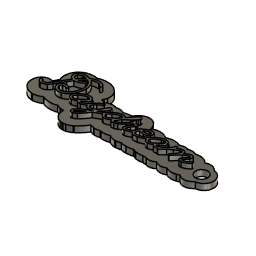
DaydreamKeyringV1 (Autodesk Fusion 360 design; units mm, degrees)
Autodesk Fusion 360 part; units mm, degrees
(part 1 of 4)
sketch "Sketch1" plane through (0, 0, 0) normal (0, 0, 1) x (1, 0, 0)
  spline S0 degree 3 poles (-17.0116, 12.697) (-15.5656, 12.5271) (-14.2829, 11.8983) (-13.2633, 10.87) knots 0 0 0 0 1 1 1 1
  line L0 (-13.2633, 10.87) -> (-13.215, 10.8207)
  line L1 (-13.215, 10.8207) -> (-13.1095, 10.7122)
  line L2 (-13.1095, 10.7122) -> (-13.0154, 10.5937)
  spline S1 degree 3 poles (-13.0154, 10.5937) (-12.1523, 9.5077) (-11.8163, 8.1682) (-12.0651, 6.8032) knots 0 0 0 0 1 1 1 1
  spline S2 degree 3 poles (-12.0651, 6.8032) (-12.1242, 6.4791) (-12.2329, 6.1392) (-12.4073, 5.8054) knots 0 0 0 0 1 1 1 1
  spline S3 degree 3 poles (-12.4073, 5.8054) (-12.5074, 5.614) (-12.6296, 5.4157) (-12.7769, 5.2205) knots 0 0 0 0 1 1 1 1
  spline S4 degree 3 poles (-12.7769, 5.2205) (-12.686, 5.1955) (-12.5953, 5.1686) (-12.505, 5.1397) knots 0 0 0 0 1 1 1 1
  spline S5 degree 3 poles (-12.505, 5.1397) (-12.3281, 5.083) (-12.1403, 5.0077) (-11.9485, 4.908) knots 0 0 0 0 1 1 1 1
  line L3 (-11.9485, 4.908) -> (-11.9101, 4.8877)
  line L4 (-11.9101, 4.8877) -> (-11.8702, 4.8661)
  spline S6 degree 3 poles (-11.8702, 4.8661) (-11.6952, 4.7703) (-11.5266, 4.6643) (-11.3653, 4.5483) knots 0 0 0 0 1 1 1 1
  spline S7 degree 3 poles (-11.3653, 4.5483) (-11.1926, 4.6617) (-11.016, 4.7697) (-10.8356, 4.8723) knots 0 0 0 0 1 1 1 1
  line L5 (-10.8356, 4.8723) -> (-10.8053, 4.8895)
  line L6 (-10.8053, 4.8895) -> (-10.7746, 4.9061)
  spline S8 degree 3 poles (-10.7746, 4.9061) (-10.3204, 5.1508) (-9.8393, 5.3371) (-9.3365, 5.4613) knots 0 0 0 0 1 1 1 1
  line L7 (-9.3365, 5.4613) -> (-9.2942, 5.4714)
  spline S9 degree 3 poles (-9.2942, 5.4714) (-8.8543, 5.5745) (-8.3289, 5.6096) (-7.7656, 5.4916) knots 0 0 0 0 1 1 1 1
  spline S10 degree 3 poles (-7.7656, 5.4916) (-7.5435, 5.4451) (-7.3065, 5.3766) (-7.0656, 5.2796) knots 0 0 0 0 1 1 1 1
  spline S11 degree 3 poles (-7.0656, 5.2796) (-7.0389, 5.2882) (-7.0121, 5.2966) (-6.985, 5.3047) knots 0 0 0 0 1 1 1 1
  spline S12 degree 3 poles (-6.985, 5.3047) (-5.8678, 5.6394) (-4.8296, 5.4328) (-4.0426, 5.0886) knots 0 0 0 0 1 1 1 1
  spline S13 degree 3 poles (-4.0426, 5.0886) (-3.921, 5.0355) (-3.7986, 4.9737) (-3.677, 4.9028) knots 0 0 0 0 1 1 1 1
  spline S14 degree 3 poles (-3.677, 4.9028) (-3.487, 4.9839) (-3.2942, 5.0598) (-3.0985, 5.1304) knots 0 0 0 0 1 1 1 1
  line L8 (-3.0985, 5.1304) -> (-3.0332, 5.1539)
  line L9 (-3.0332, 5.1539) -> (-2.9669, 5.1745)
  spline S15 degree 3 poles (-2.9669, 5.1745) (-2.2264, 5.4039) (-1.4698, 5.5072) (-0.7109, 5.4834) knots 0 0 0 0 1 1 1 1
  spline S16 degree 3 poles (-0.7109, 5.4834) (-0.4568, 5.8048) (-0.1999, 6.1247) (0.0598, 6.4431) knots 0 0 0 0 1 1 1 1
  line L10 (0.0598, 6.4431) -> (0.1573, 6.5627)
  line L11 (0.1573, 6.5627) -> (0.5924, 6.9978)
  spline S17 degree 3 poles (0.5924, 6.9978) (0.7011, 7.1065) (0.8098, 7.2152) (0.9184, 7.3239) knots 0 0 0 0 1 1 1 1
  line L12 (0.9184, 7.3239) -> (0.9577, 7.3625)
  spline S18 degree 3 poles (0.9577, 7.3625) (1.1579, 7.5569) (1.4187, 7.7663) (1.7475, 7.945) knots 0 0 0 0 1 1 1 1
  spline S19 degree 3 poles (1.7475, 7.945) (2.4822, 8.3441) (3.5755, 8.7007) (4.8203, 8.3805) knots 0 0 0 0 1 1 1 1
  spline S20 degree 3 poles (4.8203, 8.3805) (6.0538, 8.0631) (6.8371, 7.2358) (7.2909, 6.5213) knots 0 0 0 0 1 1 1 1
  line L13 (7.2909, 6.5213) -> (7.312, 6.4874)
  line L14 (7.312, 6.4874) -> (7.3319, 6.4552)
  spline S21 degree 3 poles (7.3319, 6.4552) (7.5348, 6.1216) (7.6785, 5.7617) (7.7621, 5.3924) knots 0 0 0 0 1 1 1 1
  spline S22 degree 3 poles (7.7621, 5.3924) (7.8023, 5.2143) (7.8335, 5.0337) (7.8558, 4.8512) knots 0 0 0 0 1 1 1 1
  spline S23 degree 3 poles (7.8558, 4.8512) (8.4135, 5.1588) (9.0085, 5.3986) (9.6347, 5.5692) knots 0 0 0 0 1 1 1 1
  line L15 (9.6347, 5.5692) -> (9.672, 5.5794)
  line L16 (9.672, 5.5794) -> (9.7098, 5.5886)
  spline S24 degree 3 poles (9.7098, 5.5886) (11.293, 5.9769) (12.8633, 5.6981) (14.1702, 4.7588) knots 0 0 0 0 1 1 1 1
  spline S25 degree 3 poles (14.1702, 4.7588) (14.6637, 4.9752) (15.1775, 5.1532) (15.7108, 5.2928) knots 0 0 0 0 1 1 1 1
  line L17 (15.7108, 5.2928) -> (15.8313, 5.3244)
  line L18 (15.8313, 5.3244) -> (15.9543, 5.346)
  spline S26 degree 3 poles (15.9543, 5.346) (16.9738, 5.5254) (17.9994, 5.4769) (18.9978, 5.2007) knots 0 0 0 0 1 1 1 1
  line L19 (18.9978, 5.2007) -> (19.1642, 5.1546)
  line L20 (19.1642, 5.1546) -> (19.3246, 5.0901)
  spline S27 degree 3 poles (19.3246, 5.0901) (19.4966, 5.0207) (19.6659, 4.9416) (19.8311, 4.8523) knots 0 0 0 0 1 1 1 1
  spline S28 degree 3 poles (19.8311, 4.8523) (20.051, 4.9869) (20.295, 5.1043) (20.5645, 5.1964) knots 0 0 0 0 1 1 1 1
  spline S29 degree 3 poles (20.5645, 5.1964) (21.4931, 5.5135) (22.3624, 5.406) (23.0154, 5.1941) knots 0 0 0 0 1 1 1 1
  spline S30 degree 3 poles (23.0154, 5.1941) (23.3835, 5.2965) (23.7594, 5.3726) (24.1417, 5.422) knots 0 0 0 0 1 1 1 1
  line L21 (24.1417, 5.422) -> (24.1774, 5.4264)
  spline S31 degree 3 poles (24.1774, 5.4264) (24.3442, 5.4463) (24.5277, 5.4565) (24.7241, 5.4497) knots 0 0 0 0 1 1 1 1
  line L22 (24.7241, 5.4497) -> (24.7663, 5.448)
  line L23 (24.7663, 5.448) -> (24.8398, 5.4441)
  spline S32 degree 3 poles (24.8398, 5.4441) (25.3605, 5.4125) (25.9124, 5.2986) (26.451, 5.0601) knots 0 0 0 0 1 1 1 1
  spline S33 degree 3 poles (26.451, 5.0601) (27.0557, 5.231) (27.6787, 5.313) (28.3094, 5.3117) knots 0 0 0 0 1 1 1 1
  line L24 (28.3094, 5.3117) -> (28.365, 5.3111)
  spline S34 degree 3 poles (28.365, 5.3111) (28.626, 5.3065) (28.8951, 5.2734) (29.1654, 5.2065) knots 0 0 0 0 1 1 1 1
  line L25 (29.1654, 5.2065) -> (29.223, 5.1916)
  line L26 (29.223, 5.1916) -> (29.2681, 5.1795)
  spline S35 degree 3 poles (29.2681, 5.1795) (30.2162, 4.9191) (31.3201, 4.3441) (32.0218, 3.1648) knots 0 0 0 0 1 1 1 1
  spline S36 degree 3 poles (32.0218, 3.1648) (32.1022, 3.0293) (32.1732, 2.8929) (32.2357, 2.7561) knots 0 0 0 0 1 1 1 1
  spline S37 degree 3 poles (32.2357, 2.7561) (32.8128, 2.5092) (33.2719, 2.1383) (33.616, 1.7489) knots 0 0 0 0 1 1 1 1
  line L27 (33.616, 1.7489) -> (33.6619, 1.6961)
  line L28 (33.6619, 1.6961) -> (33.6935, 1.6581)
  spline S38 degree 3 poles (33.6935, 1.6581) (34.3563, 0.8587) (34.502, -0.0325) (34.502, -0.6217) knots 0 0 0 0 1 1 1 1
  line L29 (34.502, -0.6217) -> (34.502, -1.0976)
  spline S39 degree 3 poles (34.502, -1.0976) (34.502, -1.9144) (34.2285, -2.775) (33.6258, -3.4796) knots 0 0 0 0 1 1 1 1
  spline S40 degree 3 poles (33.6258, -3.4796) (32.549, -4.7372) (31.2024, -5.649) (29.6415, -6.2002) knots 0 0 0 0 1 1 1 1
  spline S41 degree 3 poles (29.6415, -6.2002) (29.639, -6.2011) (29.6366, -6.202) (29.6338, -6.2029) knots 0 0 0 0 1 1 1 1
  spline S42 degree 3 poles (29.6338, -6.2029) (29.6313, -6.2038) (29.6285, -6.2048) (29.6256, -6.2058) knots 0 0 0 0 1 1 1 1
  spline S43 degree 3 poles (29.6256, -6.2058) (28.2575, -6.6903) (26.8147, -6.6195) (25.4936, -5.9673) knots 0 0 0 0 1 1 1 1
  spline S44 degree 3 poles (25.4936, -5.9673) (25.4542, -5.9479) (25.4145, -5.9271) (25.3735, -5.9051) knots 0 0 0 0 1 1 1 1
  spline S45 degree 3 poles (25.3735, -5.9051) (24.125, -6.7788) (22.3924, -6.8462) (21.058, -5.8602) knots 0 0 0 0 1 1 1 1
  spline S46 degree 3 poles (21.058, -5.8602) (20.2146, -6.6354) (18.8116, -7.0734) (17.5047, -6.5966) knots 0 0 0 0 1 1 1 1
  line L30 (17.5047, -6.5966) -> (17.4605, -6.5984)
  spline S47 degree 3 poles (17.4605, -6.5984) (16.9726, -6.6187) (16.4758, -6.5698) (15.9868, -6.438) knots 0 0 0 0 1 1 1 1
  spline S48 degree 3 poles (15.9868, -6.438) (15.0484, -6.7163) (14.0736, -6.7516) (13.1093, -6.5671) knots 0 0 0 0 1 1 1 1
  line L31 (13.1093, -6.5671) -> (12.9761, -6.5416)
  line L32 (12.9761, -6.5416) -> (12.8455, -6.5043)
  spline S49 degree 3 poles (12.8455, -6.5043) (12.5062, -6.4075) (12.1742, -6.277) (11.8556, -6.1104) knots 0 0 0 0 1 1 1 1
  spline S50 degree 3 poles (11.8556, -6.1104) (10.959, -6.4139) (10.0264, -6.5894) (9.0657, -6.6378) knots 0 0 0 0 1 1 1 1
  spline S51 degree 3 poles (9.0657, -6.6378) (8.3392, -6.6769) (7.6135, -6.5812) (6.922, -6.3326) knots 0 0 0 0 1 1 1 1
  spline S52 degree 3 poles (6.922, -6.3326) (6.2803, -6.5562) (5.6161, -6.707) (4.9338, -6.7845) knots 0 0 0 0 1 1 1 1
  line L33 (4.9338, -6.7845) -> (4.7783, -6.8022)
  line L34 (4.7783, -6.8022) -> (4.6218, -6.8038)
  spline S53 degree 3 poles (4.6218, -6.8038) (3.8027, -6.8123) (2.8406, -6.6275) (1.968, -6.0062) knots 0 0 0 0 1 1 1 1
  spline S54 degree 3 poles (1.968, -6.0062) (1.9586, -5.9996) (1.9493, -5.9928) (1.9401, -5.9861) knots 0 0 0 0 1 1 1 1
  spline S55 degree 3 poles (1.9401, -5.9861) (0.8662, -6.4685) (-0.2935, -6.6357) (-1.4742, -6.47) knots 0 0 0 0 1 1 1 1
  line L35 (-1.4742, -6.47) -> (-1.6858, -6.4404)
  line L36 (-1.6858, -6.4404) -> (-1.8911, -6.3814)
  spline S56 degree 3 poles (-1.8911, -6.3814) (-1.8936, -6.3807) (-1.8961, -6.38) (-1.8986, -6.3792) knots 0 0 0 0 1 1 1 1
  spline S57 degree 3 poles (-1.8986, -6.3792) (-2.6487, -6.6088) (-3.4266, -6.6988) (-4.213, -6.6578) knots 0 0 0 0 1 1 1 1
  line L37 (-4.213, -6.6578) -> (-4.3, -6.6533)
  line L38 (-4.3, -6.6533) -> (-4.3865, -6.6438)
  spline S58 degree 3 poles (-4.3865, -6.6438) (-4.8971, -6.5878) (-5.4048, -6.461) (-5.8897, -6.2522) knots 0 0 0 0 1 1 1 1
  spline S59 degree 3 poles (-5.8897, -6.2522) (-5.897, -6.2561) (-5.9044, -6.2599) (-5.9117, -6.2637) knots 0 0 0 0 1 1 1 1
  spline S60 degree 3 poles (-5.9117, -6.2637) (-6.8039, -7.6764) (-7.8863, -8.94) (-9.1522, -10.0482) knots 0 0 0 0 1 1 1 1
  line L39 (-9.1522, -10.0482) -> (-9.2488, -10.1326)
  line L40 (-9.2488, -10.1326) -> (-9.352, -10.2087)
  spline S61 degree 3 poles (-9.352, -10.2087) (-9.9808, -10.6718) (-10.6783, -11.0211) (-11.4328, -11.2431) knots 0 0 0 0 1 1 1 1
  spline S62 degree 3 poles (-11.4328, -11.2431) (-11.7998, -11.3511) (-12.1496, -11.3902) (-12.4606, -11.3902) knots 0 0 0 0 1 1 1 1
  line L41 (-12.4606, -11.3902) -> (-12.8404, -11.3902)
  spline S63 degree 3 poles (-12.8404, -11.3902) (-13.0495, -11.3902) (-13.3343, -11.3729) (-13.6596, -11.2964) knots 0 0 0 0 1 1 1 1
  spline S64 degree 3 poles (-13.6596, -11.2964) (-14.941, -10.9952) (-15.9537, -10.1675) (-16.5217, -9.0129) knots 0 0 0 0 1 1 1 1
  spline S65 degree 3 poles (-16.5217, -9.0129) (-16.6574, -8.7371) (-16.7448, -8.4674) (-16.7998, -8.221) knots 0 0 0 0 1 1 1 1
  spline S66 degree 3 poles (-16.7998, -8.221) (-16.9174, -7.6941) (-16.9595, -7.1724) (-16.9287, -6.6644) knots 0 0 0 0 1 1 1 1
  spline S67 degree 3 poles (-16.9287, -6.6644) (-17.3371, -6.6975) (-17.7496, -6.6895) (-18.1624, -6.6418) knots 0 0 0 0 1 1 1 1
  line L42 (-18.1624, -6.6418) -> (-18.2993, -6.626)
  line L43 (-18.2993, -6.626) -> (-18.4342, -6.5979)
  spline S68 degree 3 poles (-18.4342, -6.5979) (-18.9423, -6.492) (-19.4621, -6.3149) (-19.9578, -6.0404) knots 0 0 0 0 1 1 1 1
  spline S69 degree 3 poles (-19.9578, -6.0404) (-21.8163, -6.8437) (-23.8226, -6.7614) (-25.7467, -6.0039) knots 0 0 0 0 1 1 1 1
  line L44 (-25.7467, -6.0039) -> (-25.9385, -5.9284)
  line L45 (-25.9385, -5.9284) -> (-26.0235, -5.8808)
  spline S70 degree 3 poles (-26.0235, -5.8808) (-27.0239, -6.612) (-28.1898, -7.0211) (-29.451, -7.0843) knots 0 0 0 0 1 1 1 1
  line L46 (-29.451, -7.0843) -> (-29.618, -7.0926)
  line L47 (-29.618, -7.0926) -> (-29.7849, -7.0826)
  spline S71 degree 3 poles (-29.7849, -7.0826) (-31.5585, -6.9767) (-33.0924, -6.1128) (-34.0693, -4.5827) knots 0 0 0 0 1 1 1 1
  spline S72 degree 3 poles (-34.0693, -4.5827) (-34.2876, -4.2408) (-34.4452, -3.8656) (-34.537, -3.4741) knots 0 0 0 0 1 1 1 1
  spline S73 degree 3 poles (-34.537, -3.4741) (-34.6825, -2.854) (-34.729, -2.2215) (-34.6769, -1.5881) knots 0 0 0 0 1 1 1 1
  spline S74 degree 3 poles (-34.6769, -1.5881) (-34.6399, -1.1377) (-34.5131, -0.6391) (-34.2428, -0.1539) knots 0 0 0 0 1 1 1 1
  line L48 (-34.2428, -0.1539) -> (-34.2072, -0.0914)
  spline S75 degree 3 poles (-34.2072, -0.0914) (-33.8311, 0.5581) (-33.1666, 1.3164) (-32.0873, 1.6748) knots 0 0 0 0 1 1 1 1
  spline S76 degree 3 poles (-32.0873, 1.6748) (-31.2617, 1.949) (-30.4923, 1.8894) (-29.8752, 1.722) knots 0 0 0 0 1 1 1 1
  spline S77 degree 3 poles (-29.8752, 1.722) (-29.538, 2.3142) (-29.2125, 2.914) (-28.8989, 3.5214) knots 0 0 0 0 1 1 1 1
  line L49 (-28.8989, 3.5214) -> (-28.8667, 3.5837)
  line L50 (-28.8667, 3.5837) -> (-28.8316, 3.6446)
  spline S78 degree 3 poles (-28.8316, 3.6446) (-28.8105, 3.6813) (-28.7892, 3.718) (-28.768, 3.7547) knots 0 0 0 0 1 1 1 1
  spline S79 degree 3 poles (-28.768, 3.7547) (-28.8892, 3.9964) (-28.9939, 4.2524) (-29.0788, 4.5231) knots 0 0 0 0 1 1 1 1
  spline S80 degree 3 poles (-29.0788, 4.5231) (-29.4617, 5.7423) (-29.3472, 6.9455) (-29.015, 7.995) knots 0 0 0 0 1 1 1 1
  line L51 (-29.015, 7.995) -> (-28.9707, 8.1349)
  line L52 (-28.9707, 8.1349) -> (-28.9131, 8.2699)
  spline S81 degree 3 poles (-28.9131, 8.2699) (-28.4879, 9.2675) (-27.8342, 10.1832) (-26.8945, 10.8753) knots 0 0 0 0 1 1 1 1
  spline S82 degree 3 poles (-26.8945, 10.8753) (-25.9553, 11.5669) (-24.8876, 11.9194) (-23.8109, 12.0317) knots 0 0 0 0 1 1 1 1
  line L53 (-23.8109, 12.0317) -> (-23.8069, 12.0321)
  line L54 (-23.8069, 12.0321) -> (-23.8029, 12.0325)
  spline S83 degree 3 poles (-23.8029, 12.0325) (-23.0183, 12.1123) (-22.2378, 12.0846) (-21.4699, 11.9478) knots 0 0 0 0 1 1 1 1
  spline S84 degree 3 poles (-21.4699, 11.9478) (-20.7386, 12.2804) (-19.9708, 12.519) (-19.1721, 12.6612) knots 0 0 0 0 1 1 1 1
  line L55 (-19.1721, 12.6612) -> (-19.1303, 12.6684)
  spline S85 degree 3 poles (-19.1303, 12.6684) (-18.9214, 12.7031) (-18.7199, 12.7178) (-18.5296, 12.7178) knots 0 0 0 0 1 1 1 1
  line L56 (-18.5296, 12.7178) -> (-17.1886, 12.7178)
  line L57 (-17.1886, 12.7178) -> (-17.0116, 12.697)
  spline S86 degree 3 poles (-18.5843, 9.6739) (-18.1785, 9.6739) (-17.7726, 9.6739) (-17.3668, 9.6739) knots 0 0 0 0 1 1 1 1
  spline S87 degree 3 poles (-17.3668, 9.6739) (-16.5975, 9.5835) (-15.9414, 9.2588) (-15.3984, 8.6998) knots 0 0 0 0 1 1 1 1
  spline S88 degree 3 poles (-15.3984, 8.6998) (-15.0666, 8.2823) (-14.9583, 7.8088) (-15.0737, 7.2793) knots 0 0 0 0 1 1 1 1
  spline S89 degree 3 poles (-15.0737, 7.2793) (-15.2904, 6.8099) (-15.6489, 6.6543) (-16.1492, 6.8126) knots 0 0 0 0 1 1 1 1
  spline S90 degree 3 poles (-16.1492, 6.8126) (-16.2169, 6.8531) (-16.2845, 6.8937) (-16.3521, 6.9343) knots 0 0 0 0 1 1 1 1
  spline S91 degree 3 poles (-16.3521, 6.9343) (-16.4811, 7.1516) (-16.6299, 7.3546) (-16.7986, 7.5431) knots 0 0 0 0 1 1 1 1
  spline S92 degree 3 poles (-16.7986, 7.5431) (-17.3698, 7.8024) (-17.965, 7.87) (-18.5843, 7.746) knots 0 0 0 0 1 1 1 1
  spline S93 degree 3 poles (-18.5843, 7.746) (-18.7718, 7.7229) (-18.9476, 7.6688) (-19.112, 7.5837) knots 0 0 0 0 1 1 1 1
  spline S94 degree 3 poles (-19.112, 7.5837) (-18.2215, 6.7294) (-17.7142, 5.6809) (-17.59, 4.4383) knots 0 0 0 0 1 1 1 1
  spline S95 degree 3 poles (-17.59, 4.4383) (-17.5629, 3.8295) (-17.5629, 3.2207) (-17.59, 2.6119) knots 0 0 0 0 1 1 1 1
  spline S96 degree 3 poles (-17.59, 2.6119) (-17.6592, 2.0632) (-17.7539, 1.522) (-17.8741, 0.9885) knots 0 0 0 0 1 1 1 1
  spline S97 degree 3 poles (-17.8741, 0.9885) (-17.0334, 1.7098) (-16.0662, 2.1765) (-14.9722, 2.3887) knots 0 0 0 0 1 1 1 1
  spline S98 degree 3 poles (-14.9722, 2.3887) (-14.4313, 2.4525) (-13.9037, 2.3984) (-13.3894, 2.2264) knots 0 0 0 0 1 1 1 1
  spline S99 degree 3 poles (-13.3894, 2.2264) (-12.9647, 2.0117) (-12.6806, 1.6802) (-12.5371, 1.232) knots 0 0 0 0 1 1 1 1
  spline S100 degree 3 poles (-12.5371, 1.232) (-11.793, 1.252) (-11.4615, 0.8867) (-11.5427, 0.1362) knots 0 0 0 0 1 1 1 1
  spline S101 degree 3 poles (-11.5427, 0.1362) (-10.9777, 1.0123) (-10.2404, 1.7091) (-9.3308, 2.2264) knots 0 0 0 0 1 1 1 1
  spline S102 degree 3 poles (-9.3308, 2.2264) (-9.0677, 2.3681) (-8.7903, 2.4696) (-8.4988, 2.5308) knots 0 0 0 0 1 1 1 1
  spline S103 degree 3 poles (-8.4988, 2.5308) (-7.9663, 2.4609) (-7.716, 2.1565) (-7.7479, 1.6176) knots 0 0 0 0 1 1 1 1
  spline S104 degree 3 poles (-7.7479, 1.6176) (-7.7057, 1.3519) (-7.7733, 1.1219) (-7.9509, 0.9276) knots 0 0 0 0 1 1 1 1
  spline S105 degree 3 poles (-7.9509, 0.9276) (-7.9323, 0.9108) (-7.9188, 0.8905) (-7.9103, 0.8667) knots 0 0 0 0 1 1 1 1
  spline S106 degree 3 poles (-7.9103, 0.8667) (-9.1699, 0.4067) (-10.0763, -0.4321) (-10.6295, -1.6496) knots 0 0 0 0 1 1 1 1
  spline S107 degree 3 poles (-10.6295, -1.6496) (-10.5539, -1.7102) (-10.466, -1.7372) (-10.3657, -1.7308) knots 0 0 0 0 1 1 1 1
  spline S108 degree 3 poles (-10.3657, -1.7308) (-9.521, -1.5488) (-8.777, -1.1701) (-8.1335, -0.5943) knots 0 0 0 0 1 1 1 1
  spline S109 degree 3 poles (-8.1335, -0.5943) (-7.6871, 0.2174) (-7.2406, 1.0291) (-6.7942, 1.8408) knots 0 0 0 0 1 1 1 1
  spline S110 degree 3 poles (-6.7942, 1.8408) (-6.3791, 2.4405) (-5.8447, 2.5825) (-5.191, 2.2669) knots 0 0 0 0 1 1 1 1
  spline S111 degree 3 poles (-5.191, 2.2669) (-4.8735, 2.0049) (-4.7383, 1.6667) (-4.7852, 1.2523) knots 0 0 0 0 1 1 1 1
  spline S112 degree 3 poles (-4.7852, 1.2523) (-4.7831, 0.9799) (-4.817, 0.716) (-4.8866, 0.4609) knots 0 0 0 0 1 1 1 1
  spline S113 degree 3 poles (-4.8866, 0.4609) (-4.0846, 1.276) (-3.1443, 1.8781) (-2.0659, 2.2669) knots 0 0 0 0 1 1 1 1
  spline S114 degree 3 poles (-2.0659, 2.2669) (-1.4097, 2.4703) (-0.7468, 2.4974) (-0.0772, 2.3481) knots 0 0 0 0 1 1 1 1
  spline S115 degree 3 poles (-0.0772, 2.3481) (0.1305, 2.2835) (0.3267, 2.1956) (0.5113, 2.0843) knots 0 0 0 0 1 1 1 1
  spline S116 degree 3 poles (0.5113, 2.0843) (1.1286, 2.9052) (1.7644, 3.717) (2.4188, 4.5195) knots 0 0 0 0 1 1 1 1
  spline S117 degree 3 poles (2.4188, 4.5195) (2.6555, 4.7562) (2.8923, 4.993) (3.1291, 5.2297) knots 0 0 0 0 1 1 1 1
  spline S118 degree 3 poles (3.1291, 5.2297) (3.8271, 5.6416) (4.375, 5.4996) (4.7728, 4.8036) knots 0 0 0 0 1 1 1 1
  spline S119 degree 3 poles (4.7728, 4.8036) (4.9427, 4.1562) (4.8277, 3.5677) (4.4278, 3.0381) knots 0 0 0 0 1 1 1 1
  spline S120 degree 3 poles (4.4278, 3.0381) (4.8861, 2.8843) (5.116, 2.5664) (5.1178, 2.0843) knots 0 0 0 0 1 1 1 1
  spline S121 degree 3 poles (5.1178, 2.0843) (6.2434, 2.0747) (6.6829, 1.52) (6.437, 0.4203) knots 0 0 0 0 1 1 1 1
  spline S122 degree 3 poles (6.437, 0.4203) (6.3939, 0.2937) (6.3395, 0.172) (6.2746, 0.055) knots 0 0 0 0 1 1 1 1
  spline S123 degree 3 poles (6.2746, 0.055) (5.8316, -0.5466) (5.3986, -1.1554) (4.9757, -1.7713) knots 0 0 0 0 1 1 1 1
  spline S124 degree 3 poles (4.9757, -1.7713) (4.9582, -1.816) (4.9785, -1.8431) (5.0366, -1.8525) knots 0 0 0 0 1 1 1 1
  spline S125 degree 3 poles (5.0366, -1.8525) (5.6366, -1.6472) (6.2048, -1.3766) (6.7413, -1.0408) knots 0 0 0 0 1 1 1 1
  spline S126 degree 3 poles (6.7413, -1.0408) (6.8229, -0.6267) (6.965, -0.2344) (7.1675, 0.1362) knots 0 0 0 0 1 1 1 1
  spline S127 degree 3 poles (7.1675, 0.1362) (7.0741, 0.9093) (7.4191, 1.3084) (8.2024, 1.3335) knots 0 0 0 0 1 1 1 1
  spline S128 degree 3 poles (8.2024, 1.3335) (8.8283, 1.9645) (9.5726, 2.3974) (10.4347, 2.6322) knots 0 0 0 0 1 1 1 1
  spline S129 degree 3 poles (10.4347, 2.6322) (11.2987, 2.8441) (12.0496, 2.6479) (12.6872, 2.0437) knots 0 0 0 0 1 1 1 1
  spline S130 degree 3 poles (12.6872, 2.0437) (12.9575, 1.665) (13.0727, 1.2456) (13.0321, 0.7856) knots 0 0 0 0 1 1 1 1
  spline S131 degree 3 poles (13.0321, 0.7856) (13.0017, 0.5473) (12.9542, 0.3173) (12.8901, 0.0956) knots 0 0 0 0 1 1 1 1
  spline S132 degree 3 poles (12.8901, 0.0956) (13.8483, 1.2211) (15.0456, 1.972) (16.4819, 2.3481) knots 0 0 0 0 1 1 1 1
  spline S133 degree 3 poles (16.4819, 2.3481) (17.057, 2.4493) (17.6252, 2.4222) (18.1865, 2.2669) knots 0 0 0 0 1 1 1 1
  spline S134 degree 3 poles (18.1865, 2.2669) (18.674, 2.0704) (18.9987, 1.7255) (19.1606, 1.232) knots 0 0 0 0 1 1 1 1
  spline S135 degree 3 poles (19.1606, 1.232) (19.6371, 1.3023) (19.9553, 1.1129) (20.1144, 0.6638) knots 0 0 0 0 1 1 1 1
  spline S136 degree 3 poles (20.1144, 0.6638) (20.1278, 0.4744) (20.1416, 0.285) (20.1549, 0.0956) knots 0 0 0 0 1 1 1 1
  spline S137 degree 3 poles (20.1549, 0.0956) (20.4545, 0.4356) (20.7386, 0.7874) (21.0072, 1.1508) knots 0 0 0 0 1 1 1 1
  spline S138 degree 3 poles (21.0072, 1.1508) (21.0129, 1.3976) (21.0397, 1.6412) (21.0884, 1.8814) knots 0 0 0 0 1 1 1 1
  spline S139 degree 3 poles (21.0884, 1.8814) (21.3315, 2.3279) (21.6899, 2.4564) (22.1639, 2.2669) knots 0 0 0 0 1 1 1 1
  spline S140 degree 3 poles (22.1639, 2.2669) (22.252, 2.2061) (22.3397, 2.1452) (22.4278, 2.0843) knots 0 0 0 0 1 1 1 1
  spline S141 degree 3 poles (22.4278, 2.0843) (22.4927, 1.9675) (22.567, 1.8593) (22.651, 1.7596) knots 0 0 0 0 1 1 1 1
  spline S142 degree 3 poles (22.651, 1.7596) (23.2488, 2.11) (23.8913, 2.3264) (24.5788, 2.409) knots 0 0 0 0 1 1 1 1
  spline S143 degree 3 poles (24.5788, 2.409) (25.2643, 2.392) (25.7241, 2.0673) (25.9587, 1.4349) knots 0 0 0 0 1 1 1 1
  spline S144 degree 3 poles (25.9587, 1.4349) (26.6625, 2.0068) (27.4677, 2.2841) (28.3736, 2.2669) knots 0 0 0 0 1 1 1 1
  spline S145 degree 3 poles (28.3736, 2.2669) (29.3464, 2.0342) (29.732, 1.4187) (29.5303, 0.4203) knots 0 0 0 0 1 1 1 1
  spline S146 degree 3 poles (29.5303, 0.4203) (29.3549, -0.2482) (29.0371, -0.8366) (28.5765, -1.3452) knots 0 0 0 0 1 1 1 1
  spline S147 degree 3 poles (28.5765, -1.3452) (28.8456, -1.2444) (29.1025, -1.1091) (29.3476, -0.9393) knots 0 0 0 0 1 1 1 1
  spline S148 degree 3 poles (29.3476, -0.9393) (29.6707, -0.6839) (29.982, -0.4133) (30.2811, -0.1276) knots 0 0 0 0 1 1 1 1
  spline S149 degree 3 poles (30.2811, -0.1276) (30.7718, 0.1303) (31.1638, 0.0288) (31.4581, -0.432) knots 0 0 0 0 1 1 1 1
  spline S150 degree 3 poles (31.4581, -0.432) (31.4581, -0.7296) (31.4581, -1.0273) (31.4581, -1.3249) knots 0 0 0 0 1 1 1 1
  spline S151 degree 3 poles (31.4581, -1.3249) (30.7109, -2.2613) (29.764, -2.931) (28.6171, -3.3339) knots 0 0 0 0 1 1 1 1
  spline S152 degree 3 poles (28.6171, -3.3339) (27.9876, -3.5589) (27.3788, -3.5183) (26.7907, -3.2121) knots 0 0 0 0 1 1 1 1
  spline S153 degree 3 poles (26.7907, -3.2121) (26.6154, -3.0776) (26.4871, -2.9085) (26.4052, -2.7048) knots 0 0 0 0 1 1 1 1
  spline S154 degree 3 poles (26.4052, -2.7048) (26.2542, -2.0827) (26.3487, -1.501) (26.6893, -0.9596) knots 0 0 0 0 1 1 1 1
  spline S155 degree 3 poles (26.6893, -0.9596) (27.0286, -0.5461) (27.3597, -0.1267) (27.6836, 0.2985) knots 0 0 0 0 1 1 1 1
  spline S156 degree 3 poles (27.6836, 0.2985) (27.6633, 0.3121) (27.643, 0.3256) (27.6227, 0.3391) knots 0 0 0 0 1 1 1 1
  spline S157 degree 3 poles (27.6227, 0.3391) (27.098, 0.087) (26.6174, -0.2309) (26.1819, -0.6146) knots 0 0 0 0 1 1 1 1
  spline S158 degree 3 poles (26.1819, -0.6146) (25.1608, -1.6118) (24.2204, -2.6738) (23.3612, -3.8006) knots 0 0 0 0 1 1 1 1
  spline S159 degree 3 poles (23.3612, -3.8006) (22.9586, -3.4876) (22.5592, -3.1697) (22.1639, -2.8469) knots 0 0 0 0 1 1 1 1
  spline S160 degree 3 poles (22.1639, -2.8469) (22.2179, -2.7928) (22.2723, -2.7386) (22.3263, -2.6845) knots 0 0 0 0 1 1 1 1
  spline S161 degree 3 poles (22.3263, -2.6845) (22.2723, -2.6304) (22.2179, -2.5763) (22.1639, -2.5222) knots 0 0 0 0 1 1 1 1
  spline S162 degree 3 poles (22.1639, -2.5222) (22.8738, -1.7308) (23.5301, -0.8987) (24.1324, -0.0261) knots 0 0 0 0 1 1 1 1
  spline S163 degree 3 poles (24.1324, -0.0261) (24.2387, 0.1584) (24.3199, 0.3478) (24.3759, 0.5421) knots 0 0 0 0 1 1 1 1
  spline S164 degree 3 poles (24.3759, 0.5421) (23.4639, 0.1777) (22.6319, -0.3161) (21.8798, -0.9393) knots 0 0 0 0 1 1 1 1
  spline S165 degree 3 poles (21.8798, -0.9393) (21.5418, -1.2234) (21.2033, -1.5075) (20.8652, -1.7916) knots 0 0 0 0 1 1 1 1
  spline S166 degree 3 poles (20.8652, -1.7916) (20.1667, -2.5104) (19.4496, -3.2072) (18.7142, -3.8818) knots 0 0 0 0 1 1 1 1
  spline S167 degree 3 poles (18.7142, -3.8818) (18.5339, -3.7624) (18.3716, -3.6204) (18.2271, -3.4556) knots 0 0 0 0 1 1 1 1
  spline S168 degree 3 poles (18.2271, -3.4556) (17.9321, -3.491) (17.6342, -3.5248) (17.3342, -3.5571) knots 0 0 0 0 1 1 1 1
  spline S169 degree 3 poles (17.3342, -3.5571) (16.8285, -3.5781) (16.3959, -3.4158) (16.0355, -3.0701) knots 0 0 0 0 1 1 1 1
  spline S170 degree 3 poles (16.0355, -3.0701) (15.3216, -3.572) (14.5371, -3.7411) (13.6815, -3.5774) knots 0 0 0 0 1 1 1 1
  spline S171 degree 3 poles (13.6815, -3.5774) (13.0946, -3.4098) (12.6685, -3.0513) (12.4031, -2.5019) knots 0 0 0 0 1 1 1 1
  spline S172 degree 3 poles (12.4031, -2.5019) (11.3352, -3.1689) (10.1721, -3.5342) (8.9127, -3.5977) knots 0 0 0 0 1 1 1 1
  spline S173 degree 3 poles (8.9127, -3.5977) (8.1968, -3.6388) (7.588, -3.4088) (7.0863, -2.9077) knots 0 0 0 0 1 1 1 1
  spline S174 degree 3 poles (7.0863, -2.9077) (6.3148, -3.3745) (5.4828, -3.6586) (4.5901, -3.76) knots 0 0 0 0 1 1 1 1
  spline S175 degree 3 poles (4.5901, -3.76) (3.8744, -3.7675) (3.4211, -3.4293) (3.2305, -2.7454) knots 0 0 0 0 1 1 1 1
  spline S176 degree 3 poles (3.2305, -2.7454) (3.2034, -2.4207) (3.2034, -2.096) (3.2305, -1.7713) knots 0 0 0 0 1 1 1 1
  spline S177 degree 3 poles (3.2305, -1.7713) (3.2998, -1.5369) (3.3675, -1.3069) (3.4334, -1.0814) knots 0 0 0 0 1 1 1 1
  spline S178 degree 3 poles (3.4334, -1.0814) (2.705, -1.9319) (1.8459, -2.6151) (0.8562, -3.131) knots 0 0 0 0 1 1 1 1
  spline S179 degree 3 poles (0.8562, -3.131) (0.2522, -3.4411) (-0.3836, -3.5493) (-1.0513, -3.4556) knots 0 0 0 0 1 1 1 1
  spline S180 degree 3 poles (-1.0513, -3.4556) (-1.3451, -3.3713) (-1.5751, -3.2022) (-1.7412, -2.9483) knots 0 0 0 0 1 1 1 1
  spline S181 degree 3 poles (-1.7412, -2.9483) (-2.4352, -3.439) (-3.2063, -3.6622) (-4.0546, -3.618) knots 0 0 0 0 1 1 1 1
  spline S182 degree 3 poles (-4.0546, -3.618) (-4.7579, -3.5408) (-5.2787, -3.1959) (-5.6172, -2.5831) knots 0 0 0 0 1 1 1 1
  spline S183 degree 3 poles (-5.6172, -2.5831) (-6.4063, -3.0826) (-7.2247, -3.5358) (-8.0726, -3.9427) knots 0 0 0 0 1 1 1 1
  spline S184 degree 3 poles (-8.0726, -3.9427) (-8.8787, -5.3917) (-9.9069, -6.6633) (-11.1571, -7.7577) knots 0 0 0 0 1 1 1 1
  spline S185 degree 3 poles (-11.1571, -7.7577) (-11.5291, -8.0317) (-11.935, -8.2279) (-12.3747, -8.3462) knots 0 0 0 0 1 1 1 1
  spline S186 degree 3 poles (-12.3747, -8.3462) (-12.5506, -8.3462) (-12.7265, -8.3462) (-12.9023, -8.3462) knots 0 0 0 0 1 1 1 1
  spline S187 degree 3 poles (-12.9023, -8.3462) (-13.3303, -8.2638) (-13.6347, -8.0203) (-13.8155, -7.6157) knots 0 0 0 0 1 1 1 1
  spline S188 degree 3 poles (-13.8155, -7.6157) (-14.0191, -6.7795) (-13.8297, -6.049) (-13.2473, -5.4241) knots 0 0 0 0 1 1 1 1
  spline S189 degree 3 poles (-13.2473, -5.4241) (-12.546, -4.6884) (-11.7681, -4.0526) (-10.9136, -3.5165) knots 0 0 0 0 1 1 1 1
  spline S190 degree 3 poles (-10.9136, -3.5165) (-11.3951, -3.3863) (-11.774, -3.1157) (-12.05, -2.7048) knots 0 0 0 0 1 1 1 1
  spline S191 degree 3 poles (-12.05, -2.7048) (-12.7352, -3.1995) (-13.4996, -3.4836) (-14.3431, -3.5571) knots 0 0 0 0 1 1 1 1
  spline S192 degree 3 poles (-14.3431, -3.5571) (-14.8508, -3.5662) (-15.2904, -3.4038) (-15.6622, -3.0701) knots 0 0 0 0 1 1 1 1
  spline S193 degree 3 poles (-15.6622, -3.0701) (-16.3095, -3.5262) (-17.0266, -3.7088) (-17.8132, -3.618) knots 0 0 0 0 1 1 1 1
  spline S194 degree 3 poles (-17.8132, -3.618) (-18.7361, -3.4257) (-19.2705, -2.8642) (-19.4163, -1.9337) knots 0 0 0 0 1 1 1 1
  spline S195 degree 3 poles (-19.4163, -1.9337) (-20.8698, -3.5555) (-22.6083, -3.9682) (-24.6316, -3.1715) knots 0 0 0 0 1 1 1 1
  spline S196 degree 3 poles (-24.6316, -3.1715) (-25.4349, -2.7219) (-25.8881, -2.0387) (-25.9912, -1.122) knots 0 0 0 0 1 1 1 1
  spline S197 degree 3 poles (-25.9912, -1.122) (-26.3947, -1.8812) (-26.902, -2.5643) (-27.5132, -3.1715) knots 0 0 0 0 1 1 1 1
  spline S198 degree 3 poles (-27.5132, -3.1715) (-28.1026, -3.713) (-28.7993, -4.0038) (-29.6034, -4.0441) knots 0 0 0 0 1 1 1 1
  spline S199 degree 3 poles (-29.6034, -4.0441) (-30.4648, -3.9927) (-31.1141, -3.6003) (-31.5515, -2.8672) knots 0 0 0 0 1 1 1 1
  spline S200 degree 3 poles (-31.5515, -2.8672) (-31.6504, -2.4947) (-31.6775, -2.1159) (-31.6327, -1.7308) knots 0 0 0 0 1 1 1 1
  spline S201 degree 3 poles (-31.6327, -1.7308) (-31.3761, -1.1897) (-30.977, -1.0476) (-30.4354, -1.3046) knots 0 0 0 0 1 1 1 1
  spline S202 degree 3 poles (-30.4354, -1.3046) (-30.2305, -1.4635) (-30.102, -1.6732) (-30.0498, -1.9337) knots 0 0 0 0 1 1 1 1
  spline S203 degree 3 poles (-30.0498, -1.9337) (-29.8642, -2.1224) (-29.641, -2.1833) (-29.3802, -2.1163) knots 0 0 0 0 1 1 1 1
  spline S204 degree 3 poles (-29.3802, -2.1163) (-29.0021, -2.0186) (-28.6842, -1.8224) (-28.4264, -1.5278) knots 0 0 0 0 1 1 1 1
  spline S205 degree 3 poles (-28.4264, -1.5278) (-28.0974, -1.1448) (-27.7998, -0.7389) (-27.5335, -0.3102) knots 0 0 0 0 1 1 1 1
  spline S206 degree 3 poles (-27.5335, -0.3102) (-27.0664, 0.4884) (-26.62, 1.3002) (-26.1942, 2.1249) knots 0 0 0 0 1 1 1 1
  spline S207 degree 3 poles (-26.1942, 2.1249) (-25.845, 2.7309) (-25.4797, 3.3262) (-25.0984, 3.9107) knots 0 0 0 0 1 1 1 1
  spline S208 degree 3 poles (-25.0984, 3.9107) (-25.0585, 3.9618) (-25.045, 4.0159) (-25.0578, 4.073) knots 0 0 0 0 1 1 1 1
  spline S209 degree 3 poles (-25.0578, 4.073) (-26.1655, 4.7982) (-26.5172, 5.7993) (-26.113, 7.0764) knots 0 0 0 0 1 1 1 1
  spline S210 degree 3 poles (-26.113, 7.0764) (-25.6209, 8.2309) (-24.7483, 8.8735) (-23.4952, 9.0042) knots 0 0 0 0 1 1 1 1
  spline S211 degree 3 poles (-23.4952, 9.0042) (-22.6652, 9.0885) (-21.8603, 8.9871) (-21.0804, 8.6998) knots 0 0 0 0 1 1 1 1
  spline S212 degree 3 poles (-21.0804, 8.6998) (-20.3118, 9.197) (-19.4798, 9.5217) (-18.5843, 9.6739) knots 0 0 0 0 1 1 1 1
  spline S213 degree 3 poles (-23.1299, 7.1575) (-23.0209, 7.1642) (-22.9127, 7.1574) (-22.8053, 7.1372) knots 0 0 0 0 1 1 1 1
  spline S214 degree 3 poles (-22.8053, 7.1372) (-23.2151, 6.6734) (-23.5939, 6.1864) (-23.9417, 5.6762) knots 0 0 0 0 1 1 1 1
  spline S215 degree 3 poles (-23.9417, 5.6762) (-24.1932, 5.7247) (-24.4029, 5.8532) (-24.5707, 6.0617) knots 0 0 0 0 1 1 1 1
  spline S216 degree 3 poles (-24.5707, 6.0617) (-24.6235, 6.1374) (-24.6371, 6.2186) (-24.6113, 6.3052) knots 0 0 0 0 1 1 1 1
  spline S217 degree 3 poles (-24.6113, 6.3052) (-24.2485, 6.8148) (-23.7547, 7.0989) (-23.1299, 7.1575) knots 0 0 0 0 1 1 1 1
  spline S218 degree 3 poles (-19.7207, 5.5341) (-19.5157, 5.2865) (-19.3737, 5.0024) (-19.2946, 4.6818) knots 0 0 0 0 1 1 1 1
  spline S219 degree 3 poles (-19.2946, 4.6818) (-18.9575, 2.8104) (-19.3498, 1.1058) (-20.4716, -0.432) knots 0 0 0 0 1 1 1 1
  spline S220 degree 3 poles (-20.4716, -0.432) (-20.9595, -1.0309) (-21.5751, -1.43) (-22.3182, -1.6293) knots 0 0 0 0 1 1 1 1
  spline S221 degree 3 poles (-22.3182, -1.6293) (-22.9651, -1.7831) (-23.5604, -1.6749) (-24.104, -1.3046) knots 0 0 0 0 1 1 1 1
  spline S222 degree 3 poles (-24.104, -1.3046) (-24.2809, -1.1547) (-24.3891, -0.9653) (-24.4287, -0.7364) knots 0 0 0 0 1 1 1 1
  spline S223 degree 3 poles (-24.4287, -0.7364) (-24.3916, -0.5506) (-24.2834, -0.4288) (-24.104, -0.3711) knots 0 0 0 0 1 1 1 1
  spline S224 degree 3 poles (-24.104, -0.3711) (-23.9011, -0.3441) (-23.6981, -0.3441) (-23.4952, -0.3711) knots 0 0 0 0 1 1 1 1
  spline S225 degree 3 poles (-23.4952, -0.3711) (-23.1446, -0.4552) (-22.7996, -0.5567) (-22.4603, -0.6755) knots 0 0 0 0 1 1 1 1
  spline S226 degree 3 poles (-22.4603, -0.6755) (-22.1257, -0.6439) (-21.8822, -0.4816) (-21.7297, -0.1885) knots 0 0 0 0 1 1 1 1
  spline S227 degree 3 poles (-21.7297, -0.1885) (-21.4688, 0.6498) (-21.7597, 1.1706) (-22.6023, 1.3741) knots 0 0 0 0 1 1 1 1
  spline S228 degree 3 poles (-22.6023, 1.3741) (-23.2474, 1.5527) (-23.8967, 1.5933) (-24.5504, 1.4958) knots 0 0 0 0 1 1 1 1
  spline S229 degree 3 poles (-24.5504, 1.4958) (-24.12, 2.2102) (-23.6736, 2.9136) (-23.2111, 3.6063) knots 0 0 0 0 1 1 1 1
  spline S230 degree 3 poles (-23.2111, 3.6063) (-22.5662, 3.6356) (-21.9574, 3.7979) (-21.3848, 4.0933) knots 0 0 0 0 1 1 1 1
  spline S231 degree 3 poles (-21.3848, 4.0933) (-20.8437, 4.4012) (-20.3499, 4.7732) (-19.9034, 5.2094) knots 0 0 0 0 1 1 1 1
  spline S232 degree 3 poles (-19.9034, 5.2094) (-19.8317, 5.3122) (-19.7709, 5.4204) (-19.7207, 5.5341) knots 0 0 0 0 1 1 1 1
  spline S233 degree 3 poles (3.1696, 1.6785) (3.2236, 1.5591) (3.2168, 1.4374) (3.1493, 1.3132) knots 0 0 0 0 1 1 1 1
  spline S234 degree 3 poles (3.1493, 1.3132) (2.3993, 0.2083) (1.4523, -0.6846) (0.3083, -1.3655) knots 0 0 0 0 1 1 1 1
  spline S235 degree 3 poles (0.3083, -1.3655) (0.2956, -1.3083) (0.3091, -1.2542) (0.3489, -1.2031) knots 0 0 0 0 1 1 1 1
  spline S236 degree 3 poles (0.3489, -1.2031) (0.5113, -0.9596) (0.6736, -0.7161) (0.836, -0.4726) knots 0 0 0 0 1 1 1 1
  spline S237 degree 3 poles (0.836, -0.4726) (1.634, 0.2241) (2.4119, 0.9411) (3.1696, 1.6785) knots 0 0 0 0 1 1 1 1
  spline S238 degree 3 poles (10.7999, 0.8667) (10.9493, 0.8734) (11.0982, 0.8667) (11.2464, 0.8464) knots 0 0 0 0 1 1 1 1
  spline S239 degree 3 poles (11.2464, 0.8464) (10.9071, 0.6432) (10.5418, 0.5621) (10.1506, 0.6029) knots 0 0 0 0 1 1 1 1
  spline S240 degree 3 poles (10.1506, 0.6029) (10.3665, 0.7045) (10.5828, 0.7924) (10.7999, 0.8667) knots 0 0 0 0 1 1 1 1
  spline S241 degree 3 poles (-1.1325, 0.6232) (-0.9695, 0.63) (-0.8072, 0.6232) (-0.6454, 0.6029) knots 0 0 0 0 1 1 1 1
  spline S242 degree 3 poles (-0.6454, 0.6029) (-0.6138, 0.5594) (-0.6205, 0.512) (-0.6657, 0.4609) knots 0 0 0 0 1 1 1 1
  spline S243 degree 3 poles (-0.6657, 0.4609) (-1.3624, -0.4119) (-2.1944, -1.1222) (-3.1617, -1.6699) knots 0 0 0 0 1 1 1 1
  spline S244 degree 3 poles (-3.1617, -1.6699) (-3.4194, -1.7954) (-3.69, -1.836) (-3.9735, -1.7916) knots 0 0 0 0 1 1 1 1
  spline S245 degree 3 poles (-3.9735, -1.7916) (-4.0829, -1.7636) (-4.1708, -1.7027) (-4.2373, -1.609) knots 0 0 0 0 1 1 1 1
  spline S246 degree 3 poles (-4.2373, -1.609) (-4.1969, -1.4313) (-4.1157, -1.269) (-3.9938, -1.122) knots 0 0 0 0 1 1 1 1
  spline S247 degree 3 poles (-3.9938, -1.122) (-3.2092, -0.2533) (-2.2555, 0.3285) (-1.1325, 0.6232) knots 0 0 0 0 1 1 1 1
  spline S248 degree 3 poles (-14.8099, 0.5826) (-14.5724, 0.6009) (-14.3424, 0.5806) (-14.1199, 0.5218) knots 0 0 0 0 1 1 1 1
  spline S249 degree 3 poles (-14.1199, 0.5218) (-14.7067, -0.1328) (-15.3561, -0.7146) (-16.068, -1.2234) knots 0 0 0 0 1 1 1 1
  spline S250 degree 3 poles (-16.068, -1.2234) (-16.4044, -1.4661) (-16.7697, -1.6554) (-17.1638, -1.7916) knots 0 0 0 0 1 1 1 1
  spline S251 degree 3 poles (-17.1638, -1.7916) (-17.3127, -1.8187) (-17.4615, -1.8187) (-17.6103, -1.7916) knots 0 0 0 0 1 1 1 1
  spline S252 degree 3 poles (-17.6103, -1.7916) (-17.8686, -1.7202) (-17.916, -1.5781) (-17.7523, -1.3655) knots 0 0 0 0 1 1 1 1
  spline S253 degree 3 poles (-17.7523, -1.3655) (-16.9818, -0.3953) (-16.001, 0.2541) (-14.8099, 0.5826) knots 0 0 0 0 1 1 1 1
  spline S254 degree 3 poles (16.8878, 0.5826) (17.1041, 0.5826) (17.3208, 0.5826) (17.5372, 0.5826) knots 0 0 0 0 1 1 1 1
  spline S255 degree 3 poles (17.5372, 0.5826) (17.5433, 0.5399) (17.5364, 0.4994) (17.5169, 0.4609) knots 0 0 0 0 1 1 1 1
  spline S256 degree 3 poles (17.5169, 0.4609) (16.9925, -0.1177) (16.4174, -0.6385) (15.792, -1.1017) knots 0 0 0 0 1 1 1 1
  spline S257 degree 3 poles (15.792, -1.1017) (15.4738, -1.3352) (15.1357, -1.5382) (14.7773, -1.7105) knots 0 0 0 0 1 1 1 1
  spline S258 degree 3 poles (14.7773, -1.7105) (14.4774, -1.8416) (14.1799, -1.8416) (13.8844, -1.7105) knots 0 0 0 0 1 1 1 1
  spline S259 degree 3 poles (13.8844, -1.7105) (13.8406, -1.6404) (13.8341, -1.566) (13.8642, -1.4872) knots 0 0 0 0 1 1 1 1
  spline S260 degree 3 poles (13.8642, -1.4872) (14.4896, -0.6321) (15.2944, -0.0031) (16.279, 0.4) knots 0 0 0 0 1 1 1 1
  spline S261 degree 3 poles (16.279, 0.4) (16.4852, 0.4682) (16.6881, 0.5291) (16.8878, 0.5826) knots 0 0 0 0 1 1 1 1
  spline S262 degree 3 poles (11.0029, -1.2031) (10.1648, -1.6806) (9.2719, -1.8362) (8.3242, -1.6699) knots 0 0 0 0 1 1 1 1
  spline S263 degree 3 poles (8.3242, -1.6699) (8.2804, -1.6399) (8.2532, -1.5993) (8.243, -1.5481) knots 0 0 0 0 1 1 1 1
  spline S264 degree 3 poles (8.243, -1.5481) (8.2901, -1.4061) (8.3376, -1.264) (8.3851, -1.122) knots 0 0 0 0 1 1 1 1
  spline S265 degree 3 poles (8.3851, -1.122) (8.4127, -1.0386) (8.4602, -0.9709) (8.5271, -0.919) knots 0 0 0 0 1 1 1 1
  spline S266 degree 3 poles (8.5271, -0.919) (9.3271, -1.2303) (10.1522, -1.325) (11.0029, -1.2031) knots 0 0 0 0 1 1 1 1
  spline S267 degree 3 poles (-18.5032, 9.5115) (-17.6451, 9.5873) (-16.8334, 9.4317) (-16.068, 9.0448) knots 0 0 0 0 1 1 1 1
  spline S268 degree 3 poles (-16.068, 9.0448) (-15.7039, 8.7886) (-15.4265, 8.4572) (-15.236, 8.0504) knots 0 0 0 0 1 1 1 1
  spline S269 degree 3 poles (-15.236, 8.0504) (-15.2004, 7.7765) (-15.2139, 7.5059) (-15.2766, 7.2387) knots 0 0 0 0 1 1 1 1
  spline S270 degree 3 poles (-15.2766, 7.2387) (-15.5068, 6.9229) (-15.7976, 6.8485) (-16.1492, 7.0155) knots 0 0 0 0 1 1 1 1
  spline S271 degree 3 poles (-16.1492, 7.0155) (-16.298, 7.2184) (-16.4468, 7.4213) (-16.5956, 7.6243) knots 0 0 0 0 1 1 1 1
  spline S272 degree 3 poles (-16.5956, 7.6243) (-16.7827, 7.7516) (-16.9856, 7.8463) (-17.2044, 7.9084) knots 0 0 0 0 1 1 1 1
  spline S273 degree 3 poles (-17.2044, 7.9084) (-17.8327, 8.0074) (-18.455, 7.9803) (-19.0714, 7.8272) knots 0 0 0 0 1 1 1 1
  spline S274 degree 3 poles (-19.0714, 7.8272) (-19.2136, 7.8005) (-19.3354, 7.7397) (-19.4366, 7.6446) knots 0 0 0 0 1 1 1 1
  spline S275 degree 3 poles (-19.4366, 7.6446) (-18.2597, 6.6022) (-17.6915, 5.2899) (-17.732, 3.7077) knots 0 0 0 0 1 1 1 1
  spline S276 degree 3 poles (-17.732, 3.7077) (-17.7278, 2.969) (-17.8022, 2.2384) (-17.9553, 1.5161) knots 0 0 0 0 1 1 1 1
  spline S277 degree 3 poles (-17.9553, 1.5161) (-18.065, 1.1333) (-18.1732, 0.7545) (-18.2799, 0.3797) knots 0 0 0 0 1 1 1 1
  spline S278 degree 3 poles (-18.2799, 0.3797) (-17.3485, 1.3234) (-16.2324, 1.9389) (-14.9316, 2.2264) knots 0 0 0 0 1 1 1 1
  spline S279 degree 3 poles (-14.9316, 2.2264) (-14.4322, 2.2789) (-13.9451, 2.2248) (-13.4705, 2.064) knots 0 0 0 0 1 1 1 1
  spline S280 degree 3 poles (-13.4705, 2.064) (-13.0012, 1.8358) (-12.7239, 1.4638) (-12.6385, 0.9479) knots 0 0 0 0 1 1 1 1
  spline S281 degree 3 poles (-12.6385, 0.9479) (-12.2929, 1.1485) (-12.0088, 1.0809) (-11.7862, 0.745) knots 0 0 0 0 1 1 1 1
  spline S282 degree 3 poles (-11.7862, 0.745) (-11.7369, 0.5501) (-11.7166, 0.3539) (-11.7253, 0.1565) knots 0 0 0 0 1 1 1 1
  spline S283 degree 3 poles (-11.7253, 0.1565) (-11.7412, 0.0275) (-11.7885, -0.0874) (-11.8674, -0.1885) knots 0 0 0 0 1 1 1 1
  spline S284 degree 3 poles (-11.8674, -0.1885) (-12.6906, -0.687) (-13.4685, -1.2485) (-14.2011, -1.8728) knots 0 0 0 0 1 1 1 1
  spline S285 degree 3 poles (-14.2011, -1.8728) (-13.5929, -1.7379) (-13.0382, -1.4809) (-12.5371, -1.1017) knots 0 0 0 0 1 1 1 1
  spline S286 degree 3 poles (-12.5371, -1.1017) (-12.2462, -0.8649) (-11.9553, -0.6282) (-11.6645, -0.3914) knots 0 0 0 0 1 1 1 1
  spline S287 degree 3 poles (-11.6645, -0.3914) (-11.0097, 0.8181) (-10.0559, 1.7042) (-8.8032, 2.2669) knots 0 0 0 0 1 1 1 1
  spline S288 degree 3 poles (-8.8032, 2.2669) (-8.4055, 2.4163) (-8.1146, 2.3013) (-7.9306, 1.922) knots 0 0 0 0 1 1 1 1
  spline S289 degree 3 poles (-7.9306, 1.922) (-7.9035, 1.7055) (-7.9035, 1.489) (-7.9306, 1.2726) knots 0 0 0 0 1 1 1 1
  spline S290 degree 3 poles (-7.9306, 1.2726) (-7.9736, 1.1483) (-8.048, 1.0469) (-8.1538, 0.9682) knots 0 0 0 0 1 1 1 1
  spline S291 degree 3 poles (-8.1538, 0.9682) (-9.4037, 0.4623) (-10.2899, -0.4103) (-10.8122, -1.6496) knots 0 0 0 0 1 1 1 1
  spline S292 degree 3 poles (-10.8122, -1.6496) (-10.8439, -1.7082) (-10.8371, -1.7623) (-10.7919, -1.8119) knots 0 0 0 0 1 1 1 1
  spline S293 degree 3 poles (-10.7919, -1.8119) (-10.4542, -1.9174) (-10.116, -1.9107) (-9.7772, -1.7916) knots 0 0 0 0 1 1 1 1
  spline S294 degree 3 poles (-9.7772, -1.7916) (-9.1587, -1.5502) (-8.5905, -1.2255) (-8.0726, -0.8176) knots 0 0 0 0 1 1 1 1
  spline S295 degree 3 poles (-8.0726, -0.8176) (-7.5769, 0.0316) (-7.0967, 0.8907) (-6.6318, 1.7596) knots 0 0 0 0 1 1 1 1
  spline S296 degree 3 poles (-6.6318, 1.7596) (-6.2789, 2.2687) (-5.8257, 2.3836) (-5.2722, 2.1046) knots 0 0 0 0 1 1 1 1
  spline S297 degree 3 poles (-5.2722, 2.1046) (-5.0163, 1.8781) (-4.9216, 1.594) (-4.9881, 1.2523) knots 0 0 0 0 1 1 1 1
  spline S298 degree 3 poles (-4.9881, 1.2523) (-4.9558, 0.9286) (-5.0166, 0.6242) (-5.1707, 0.3391) knots 0 0 0 0 1 1 1 1
  spline S299 degree 3 poles (-5.1707, 0.3391) (-5.4534, -0.1602) (-5.7984, -0.6134) (-6.2057, -1.0205) knots 0 0 0 0 1 1 1 1
  spline S300 degree 3 poles (-6.2057, -1.0205) (-5.6811, -0.7804) (-5.2685, -0.4084) (-4.9678, 0.0956) knots 0 0 0 0 1 1 1 1
  spline S301 degree 3 poles (-4.9678, 0.0956) (-4.0788, 1.1049) (-2.9898, 1.8017) (-1.7007, 2.1858) knots 0 0 0 0 1 1 1 1
  spline S302 degree 3 poles (-1.7007, 2.1858) (-1.187, 2.2649) (-0.6729, 2.2649) (-0.1584, 2.1858) knots 0 0 0 0 1 1 1 1
  spline S303 degree 3 poles (-0.1584, 2.1858) (0.1115, 2.1152) (0.3482, 1.9866) (0.5519, 1.8002) knots 0 0 0 0 1 1 1 1
  spline S304 degree 3 poles (0.5519, 1.8002) (1.2493, 2.7349) (1.9663, 3.6548) (2.7029, 4.56) knots 0 0 0 0 1 1 1 1
  spline S305 degree 3 poles (2.7029, 4.56) (2.9493, 4.8743) (3.2536, 5.1111) (3.6161, 5.2703) knots 0 0 0 0 1 1 1 1
  spline S306 degree 3 poles (3.6161, 5.2703) (4.078, 5.3268) (4.4095, 5.1441) (4.6104, 4.7224) knots 0 0 0 0 1 1 1 1
  spline S307 degree 3 poles (4.6104, 4.7224) (4.7504, 4.0088) (4.5678, 3.3932) (4.0625, 2.8757) knots 0 0 0 0 1 1 1 1
  spline S308 degree 3 poles (4.0625, 2.8757) (4.6774, 2.8629) (4.9885, 2.545) (4.996, 1.922) knots 0 0 0 0 1 1 1 1
  spline S309 degree 3 poles (4.996, 1.922) (6.1074, 1.9674) (6.5202, 1.4533) (6.234, 0.3797) knots 0 0 0 0 1 1 1 1
  spline S310 degree 3 poles (6.234, 0.3797) (6.1224, 0.17) (6.0007, -0.0329) (5.8686, -0.2291) knots 0 0 0 0 1 1 1 1
  spline S311 degree 3 poles (5.8686, -0.2291) (5.3671, -0.8055) (4.941, -1.4346) (4.5901, -2.1163) knots 0 0 0 0 1 1 1 1
  spline S312 degree 3 poles (4.5901, -2.1163) (4.6239, -2.1231) (4.6578, -2.1298) (4.6916, -2.1366) knots 0 0 0 0 1 1 1 1
  spline S313 degree 3 poles (4.6916, -2.1366) (5.4853, -1.9223) (6.2296, -1.5976) (6.924, -1.1626) knots 0 0 0 0 1 1 1 1
  spline S314 degree 3 poles (6.924, -1.1626) (6.978, -0.7298) (7.1131, -0.324) (7.3298, 0.055) knots 0 0 0 0 1 1 1 1
  spline S315 degree 3 poles (7.3298, 0.055) (7.3432, 0.2715) (7.3566, 0.488) (7.3704, 0.7044) knots 0 0 0 0 1 1 1 1
  spline S316 degree 3 poles (7.3704, 0.7044) (7.5531, 1.0359) (7.8303, 1.1644) (8.2024, 1.09) knots 0 0 0 0 1 1 1 1
  spline S317 degree 3 poles (8.2024, 1.09) (8.8969, 1.8162) (9.7358, 2.2897) (10.7188, 2.5105) knots 0 0 0 0 1 1 1 1
  spline S318 degree 3 poles (10.7188, 2.5105) (11.4696, 2.6165) (12.0987, 2.3933) (12.606, 1.8408) knots 0 0 0 0 1 1 1 1
  spline S319 degree 3 poles (12.606, 1.8408) (13.0796, 0.8063) (12.843, -0.0257) (11.8957, -0.6552) knots 0 0 0 0 1 1 1 1
  spline S320 degree 3 poles (11.8957, -0.6552) (11.2326, -0.9989) (10.5292, -1.1342) (9.7853, -1.0611) knots 0 0 0 0 1 1 1 1
  spline S321 degree 3 poles (9.7853, -1.0611) (9.3181, -0.9645) (8.8579, -0.8563) (8.4054, -0.7364) knots 0 0 0 0 1 1 1 1
  spline S322 degree 3 poles (8.4054, -0.7364) (8.1972, -1.0225) (8.0957, -1.3404) (8.101, -1.6902) knots 0 0 0 0 1 1 1 1
  spline S323 degree 3 poles (8.101, -1.6902) (8.1793, -1.7959) (8.2808, -1.8703) (8.4054, -1.9134) knots 0 0 0 0 1 1 1 1
  spline S324 degree 3 poles (8.4054, -1.9134) (9.3482, -1.9956) (10.2411, -1.8197) (11.084, -1.3858) knots 0 0 0 0 1 1 1 1
  spline S325 degree 3 poles (11.084, -1.3858) (11.5982, -1.1289) (12.0853, -0.8312) (12.5451, -0.4929) knots 0 0 0 0 1 1 1 1
  spline S326 degree 3 poles (12.5451, -0.4929) (12.9489, -0.0892) (13.3548, 0.3166) (13.7627, 0.7247) knots 0 0 0 0 1 1 1 1
  spline S327 degree 3 poles (13.7627, 0.7247) (14.6402, 1.495) (15.6548, 1.9955) (16.8066, 2.2264) knots 0 0 0 0 1 1 1 1
  spline S328 degree 3 poles (16.8066, 2.2264) (17.5408, 2.3467) (18.1837, 2.164) (18.7344, 1.6785) knots 0 0 0 0 1 1 1 1
  spline S329 degree 3 poles (18.7344, 1.6785) (18.8927, 1.4703) (19.0076, 1.2403) (19.0794, 0.9885) knots 0 0 0 0 1 1 1 1
  spline S330 degree 3 poles (19.0794, 0.9885) (19.4236, 1.1379) (19.7008, 1.0567) (19.9114, 0.745) knots 0 0 0 0 1 1 1 1
  spline S331 degree 3 poles (19.9114, 0.745) (19.9386, 0.488) (19.9386, 0.2309) (19.9114, -0.0261) knots 0 0 0 0 1 1 1 1
  spline S332 degree 3 poles (19.9114, -0.0261) (19.8842, -0.0802) (19.8575, -0.1344) (19.8303, -0.1885) knots 0 0 0 0 1 1 1 1
  spline S333 degree 3 poles (19.8303, -0.1885) (19.0072, -0.687) (18.2291, -1.2485) (17.4966, -1.8728) knots 0 0 0 0 1 1 1 1
  spline S334 degree 3 poles (17.4966, -1.8728) (17.9268, -1.7799) (18.3326, -1.6175) (18.7142, -1.3858) knots 0 0 0 0 1 1 1 1
  spline S335 degree 3 poles (18.7142, -1.3858) (19.7511, -0.7412) (20.5831, 0.1043) (21.2102, 1.1508) knots 0 0 0 0 1 1 1 1
  spline S336 degree 3 poles (21.2102, 1.1508) (21.2236, 1.3673) (21.2374, 1.5838) (21.2508, 1.8002) knots 0 0 0 0 1 1 1 1
  spline S337 degree 3 poles (21.2508, 1.8002) (21.4638, 2.1794) (21.7682, 2.2674) (22.1639, 2.064) knots 0 0 0 0 1 1 1 1
  spline S338 degree 3 poles (22.1639, 2.064) (22.3421, 1.9036) (22.4639, 1.7074) (22.5292, 1.4755) knots 0 0 0 0 1 1 1 1
  spline S339 degree 3 poles (22.5292, 1.4755) (22.9996, 1.7649) (23.5004, 1.9881) (24.0309, 2.1452) knots 0 0 0 0 1 1 1 1
  spline S340 degree 3 poles (24.0309, 2.1452) (24.634, 2.3293) (25.1547, 2.2008) (25.5934, 1.7596) knots 0 0 0 0 1 1 1 1
  spline S341 degree 3 poles (25.5934, 1.7596) (25.7363, 1.5816) (25.8106, 1.3787) (25.8167, 1.1508) knots 0 0 0 0 1 1 1 1
  spline S342 degree 3 poles (25.8167, 1.1508) (26.0334, 1.2515) (26.2363, 1.38) (26.4255, 1.5364) knots 0 0 0 0 1 1 1 1
  spline S343 degree 3 poles (26.4255, 1.5364) (27.0371, 1.9644) (27.7136, 2.1403) (28.4547, 2.064) knots 0 0 0 0 1 1 1 1
  spline S344 degree 3 poles (28.4547, 2.064) (28.8675, 1.9758) (29.1585, 1.739) (29.3273, 1.3538) knots 0 0 0 0 1 1 1 1
  spline S345 degree 3 poles (29.3273, 1.3538) (29.3736, 0.9148) (29.3464, 0.4819) (29.2462, 0.055) knots 0 0 0 0 1 1 1 1
  spline S346 degree 3 poles (29.2462, 0.055) (28.9304, -0.5905) (28.5245, -1.1723) (28.0286, -1.6902) knots 0 0 0 0 1 1 1 1
  spline S347 degree 3 poles (28.0286, -1.6902) (28.0046, -1.7301) (28.018, -1.7571) (28.0692, -1.7713) knots 0 0 0 0 1 1 1 1
  spline S348 degree 3 poles (28.0692, -1.7713) (28.9422, -1.4804) (29.693, -1.0001) (30.3217, -0.3305) knots 0 0 0 0 1 1 1 1
  spline S349 degree 3 poles (30.3217, -0.3305) (30.6569, -0.0695) (30.9613, -0.1033) (31.2349, -0.432) knots 0 0 0 0 1 1 1 1
  spline S350 degree 3 poles (31.2349, -0.432) (31.3148, -0.7421) (31.3148, -1.0533) (31.2349, -1.3655) knots 0 0 0 0 1 1 1 1
  spline S351 degree 3 poles (31.2349, -1.3655) (30.3785, -2.3167) (29.3302, -2.9458) (28.0895, -3.2527) knots 0 0 0 0 1 1 1 1
  spline S352 degree 3 poles (28.0895, -3.2527) (26.7376, -3.3584) (26.2574, -2.7563) (26.6487, -1.4467) knots 0 0 0 0 1 1 1 1
  spline S353 degree 3 poles (26.6487, -1.4467) (26.7363, -1.244) (26.8447, -1.0546) (26.9734, -0.8785) knots 0 0 0 0 1 1 1 1
  spline S354 degree 3 poles (26.9734, -0.8785) (27.3922, -0.4191) (27.7644, 0.0747) (28.0895, 0.6029) knots 0 0 0 0 1 1 1 1
  spline S355 degree 3 poles (28.0895, 0.6029) (27.9056, 0.6327) (27.7299, 0.6056) (27.5619, 0.5218) knots 0 0 0 0 1 1 1 1
  spline S356 degree 3 poles (27.5619, 0.5218) (26.9372, 0.2095) (26.369, -0.1828) (25.8572, -0.6552) knots 0 0 0 0 1 1 1 1
  spline S357 degree 3 poles (25.8572, -0.6552) (24.9359, -1.5624) (24.0905, -2.5297) (23.3206, -3.5571) knots 0 0 0 0 1 1 1 1
  spline S358 degree 3 poles (23.3206, -3.5571) (23.0227, -3.32) (22.7321, -3.0765) (22.448, -2.8266) knots 0 0 0 0 1 1 1 1
  spline S359 degree 3 poles (22.448, -2.8266) (22.4886, -2.7725) (22.5292, -2.7183) (22.5698, -2.6642) knots 0 0 0 0 1 1 1 1
  spline S360 degree 3 poles (22.5698, -2.6642) (22.5032, -2.6068) (22.4696, -2.5391) (22.4683, -2.4613) knots 0 0 0 0 1 1 1 1
  spline S361 degree 3 poles (22.4683, -2.4613) (23.1238, -1.7114) (23.7326, -0.9268) (24.2947, -0.1073) knots 0 0 0 0 1 1 1 1
  spline S362 degree 3 poles (24.2947, -0.1073) (24.4554, 0.1597) (24.5703, 0.4438) (24.6397, 0.745) knots 0 0 0 0 1 1 1 1
  spline S363 degree 3 poles (24.6397, 0.745) (24.416, 0.7314) (24.1997, 0.684) (23.9903, 0.6029) knots 0 0 0 0 1 1 1 1
  spline S364 degree 3 poles (23.9903, 0.6029) (22.8843, 0.0435) (21.8697, -0.6465) (20.9464, -1.4669) knots 0 0 0 0 1 1 1 1
  spline S365 degree 3 poles (20.9464, -1.4669) (20.1959, -2.1834) (19.452, -2.9071) (18.7142, -3.6383) knots 0 0 0 0 1 1 1 1
  spline S366 degree 3 poles (18.7142, -3.6383) (18.5583, -3.4617) (18.3757, -3.3263) (18.1662, -3.2324) knots 0 0 0 0 1 1 1 1
  spline S367 degree 3 poles (18.1662, -3.2324) (17.6902, -3.3629) (17.21, -3.3832) (16.7254, -3.2933) knots 0 0 0 0 1 1 1 1
  spline S368 degree 3 poles (16.7254, -3.2933) (16.4588, -3.2073) (16.2421, -3.0517) (16.0761, -2.8266) knots 0 0 0 0 1 1 1 1
  spline S369 degree 3 poles (16.0761, -2.8266) (15.4344, -3.2947) (14.7177, -3.5044) (13.925, -3.4556) knots 0 0 0 0 1 1 1 1
  spline S370 degree 3 poles (13.925, -3.4556) (13.4303, -3.3525) (13.0313, -3.1022) (12.7278, -2.7048) knots 0 0 0 0 1 1 1 1
  spline S371 degree 3 poles (12.7278, -2.7048) (12.6596, -2.5412) (12.5719, -2.3923) (12.4639, -2.2584) knots 0 0 0 0 1 1 1 1
  spline S372 degree 3 poles (12.4639, -2.2584) (11.5991, -2.7969) (10.6656, -3.1554) (9.6635, -3.3339) knots 0 0 0 0 1 1 1 1
  spline S373 degree 3 poles (9.6635, -3.3339) (9.1493, -3.4151) (8.6351, -3.4151) (8.1213, -3.3339) knots 0 0 0 0 1 1 1 1
  spline S374 degree 3 poles (8.1213, -3.3339) (7.732, -3.2106) (7.4005, -3.0009) (7.1269, -2.7048) knots 0 0 0 0 1 1 1 1